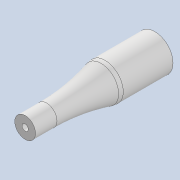
# Autodesk Inventor part: needle_conn_1
Saved by Autodesk Inventor 2020 (Build 240168000, 168)
## iProperties
Created: 2021-07-15
Part Number: needle_conn_1
Material: Generic
Document SubType Name: Modeling
Designer: Shuang Peng
Density: 1 g/cm^3
Appearance: Default
Author: Shuang Peng
Autodesk Inventor part; units mm, degrees
ref_plane "YZ Plane" through (0, 0, 0) normal (1, 0, 0) x (0, 1, 0)
ref_plane "XZ Plane" through (0, 0, 0) normal (0, 1, 0) x (-1, 0, 0)
ref_plane "XY Plane" through (0, 0, 0) normal (0, 0, 1) x (1, 0, 0)
sketch "Sketch1" plane through (0, 0, 0) normal (0, 0, 1) x (1, 0, 0)
  circle A0 centre (0, -6.4566) radius 1.5 projected
  circle A1 centre (0, -6.4566) radius 1.5
  circle A2 centre (0, -6.4566) radius 3.5
  point P0 (0, 0)
  dimension "d0" = 3
  dimension "d1" = 7
  constraints: 2 centre point, 2 coincident
  measures "d0" diameter of A1
  measures "d1" diameter of A2
extrude "Extrusion1" add sketch "Sketch1" along normal blind 8
sketch "Sketch2" plane through (0, -6.4566, 8) normal (0, 0, 1) x (1, 0, 0)
  circle A0 centre (0, 0) radius 3.5 projected
  point P0 (0, 6.4566)
extrude "Extrusion2" add sketch "Sketch2" along normal blind 2
sketch "Sketch3" plane through (0, -6.4566, 10) normal (0, 0, 1) x (1, 0, 0)
  circle A0 centre (0, 0) radius 3.5 projected
  circle A1 centre (0, 0) radius 0.6
  circle A2 centre (0, 0) radius 2
  point P0 (0, 6.4566)
  dimension "d6" = 1.2
  dimension "d7" = 4
  constraints: 2 centre point, 2 coincident
  measures "d6" diameter of A1
  measures "d7" diameter of A2
extrude "Extrusion3" add sketch "Sketch3" along normal blind 15 contours A2
fillet "Fillet1" radius 40 1 edges at (-2, -6.4566, 10)
fillet "Fillet2" radius 3 1 edges at (-3.5, -6.4566, 10)
chamfer "Chamfer1" distance 0.5 angle 45 1 edges at (-1.5, -6.4566, 0)
chamfer "Chamfer2" distance 0.5 angle 45 1 edges at (-2, -6.4566, 25)
body "Solid1"
